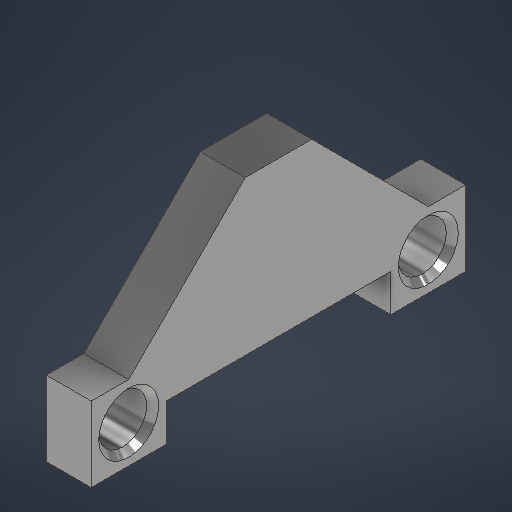
# Autodesk Inventor part: stopka
Saved by Autodesk Inventor 2026.1 (Build 301233020, 233B)
## iProperties
Created: 2025-11-09
Part Number: stopka
Material: Steel, High Strength, Low Alloy
Document SubType Name: Modeling
Designer: Jan
Density: 7.85 g/cm^3
Appearance: Steel - Polished
Author: Jan
Autodesk Inventor part; units mm, degrees
ref_plane "YZ Plane" through (0, 0, 0) normal (1, 0, 0) x (0, 1, 0)
ref_plane "XZ Plane" through (0, 0, 0) normal (0, 1, 0) x (-1, 0, 0)
ref_plane "XY Plane" through (0, 0, 0) normal (0, 0, 1) x (1, 0, 0)
sketch "Sketch1" plane through (0, 0, 0) normal (1, 0, 0) x (0, 1, 0)
  line L0 (-1, 7.5) -> (-6, 7.5)
  line L1 (-6, 7.5) -> (-6, 12.5)
  line L2 (-6, 12.5) -> (-1, 12.5)
  line L3 (-1, 12.5) -> (-1, 7.5)
  circle A0 centre (-3.5, 10) radius 1.6
  line L4 (-3.5, 7.5) -> (0.277, 7.5) construction
  line L5 (-3.5, 7.5) -> (0.0775, 7.5) construction
  line L6 (-1, 10) -> (6.7782, 2.2218)
  line L7 (-1, 10) -> (10, 10) construction
  line L8 (6.7782, 2.2218) -> (6.7782, -1.9926)
  line L9 (-3.5, 7.5) -> (-3.5, 7.5)
  line L10 (-3.5, 7.5) -> (-3.5, 7.5) construction
  line L11 (-3.5, 7.5) -> (-3.5, 4.25)
  line L12 (3.8235, 0) -> (5.1347, 0) construction
  line L13 (-1, -7.5) -> (-6, -7.5)
  line L14 (-6, -7.5) -> (-6, -12.5)
  line L15 (-6, -12.5) -> (-1, -12.5)
  line L16 (-1, -12.5) -> (-1, -7.5)
  circle A1 centre (-3.5, -10) radius 1.6
  line L17 (-3.5, -7.5) -> (0.277, -7.5) construction
  line L18 (-3.5, -7.5) -> (0.0775, -7.5) construction
  line L19 (-1, -10) -> (6.7782, -2.2218)
  line L20 (-1, -10) -> (10, -10) construction
  line L21 (6.7782, -2.2218) -> (6.7782, -1.9926)
  line L22 (-3.5, -7.5) -> (-3.5, -7.5)
  line L23 (-3.5, -7.5) -> (-3.5, -7.5) construction
  line L24 (-3.5, -7.5) -> (-3.5, 4.25)
  point P0 (0, 0)
  point P1 (-3.5, 12.5)
  point P2 (-3.5, -12.5)
  dimension "d0" = 5
  dimension "d1" = 5
  dimension "d2" = 7.5
  dimension "d3" = 1
  dimension "d4" = 3.2
  dimension "d5" = 2.5
  dimension "d6" = 2.5
  dimension "d7" = 10
  dimension "d10" = 11
  dimension "d11" = 45
  dimension "d12" = 45
  dimension "d14" = 3.25
  dimension "d15" = 2.5
  constraints: 50 end point, 14 symmetric about line, 6 horizontal, 3 midpoint, 2 centre point, 2 equal length, 2 parallel, 2 vertical, 1 perpendicular, 1 other
  measures "d0" distance of L1.end L2.end
  measures "d1" distance of L0.end L1.end
  measures "d2" vertical distance of point (0, 0) L0.end
  measures "d3" horizontal distance of point (0, 0) L2.end
  measures "d4" diameter of A0
  measures "d5" distance from line of L1 A0.centre
  measures "d6" distance of point (-3.5, 12.5) A0.centre
  measures "d7" vertical distance of point (0, 0) A0.centre
  measures "d10" distance of L6.start L6.end
  measures "d11" angle of L6 L7
  measures "d12" angle of L9 L10
  measures "d14" distance of L9.end L11.end
  measures "d15" distance from line of L0.end L11
extrude "Extrusion1" add sketch "Sketch1" along normal blind 3
chamfer "Chamfer1" distance 0.4 angle 45 2 edges at (3, -5.1, 10) (3, -5.1, -10)
equation "\"d0\" = d1"
equation "\"d5\" = 0.5 * d0"
equation "\"d6\" = d5"
body "Solid1"
